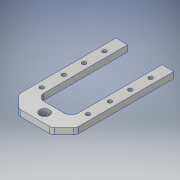
# Autodesk Inventor part: Part1_new1
Saved by Autodesk Inventor 2016 (Build 200138000, 138)
## iProperties
Created: 2017-01-04
Part Number: Part1_new1
Material: Aluminium 6061
Document SubType Name: Modeling
Designer: Marc
Density: 2.7 g/cm^3
Appearance: Aluminium - flach
Mass: 11.4747 g
Surface Area: 37.37 cm^2
Volume: 4.24988 cm^3
Author: Marc
Autodesk Inventor part; units mm, degrees
ref_plane "YZ Plane" through (0, 0, 0) normal (1, 0, 0) x (0, 1, 0)
ref_plane "XZ Plane" through (0, 0, 0) normal (0, 1, 0) x (-1, 0, 0)
ref_plane "XY Plane" through (0, 0, 0) normal (0, 0, 1) x (1, 0, 0)
sketch "Skizze2" plane through (0, 0, 0) normal (0, 0, 1) x (1, 0, 0)
  line L0 (-26.1954, 0) -> (26.1954, 0) projected
  line L1 (0, -30.2532) -> (0, 68.0422) projected
  line L2 (-18.5, 54) -> (-18.5, -6.7574)
  line L3 (-9.2574, -16) -> (9.2574, -16)
  line L4 (18.5, -6.7574) -> (18.5, 54)
  line L5 (18.5, 54) -> (11, 54)
  line L6 (11, 54) -> (11, 3)
  line L7 (-11, 3) -> (-11, 54)
  line L8 (-11, 54) -> (-18.5, 54)
  circle A0 centre (0, -10) radius 3.15
  circle A1 centre (-14.75, 43) radius 1.3
  circle A2 centre (-14.75, 30) radius 1.3
  circle A3 centre (-14.75, 17) radius 1.3
  circle A4 centre (-14.75, 3) radius 1.3
  circle A5 centre (14.75, 43) radius 1.3
  circle A6 centre (14.75, 30) radius 1.3
  circle A7 centre (14.75, 17) radius 1.3
  circle A8 centre (14.75, 3) radius 1.3
  line L9 (-17.6213, -8.8787) -> (-11.3787, -15.1213)
  line L10 (11.3787, -15.1213) -> (17.6213, -8.8787)
  arc A9 (-18.5, -6.7574) -> (-17.6213, -8.8787) centre (-15.5, -6.7574) ccw
  arc A10 (-11.3787, -15.1213) -> (-9.2574, -16) centre (-9.2574, -13) ccw
  arc A11 (9.2574, -16) -> (11.3787, -15.1213) centre (9.2574, -13) ccw
  line L11 (-11, 3) -> (-11, 0.2426)
  line L12 (11, 3) -> (11, 0.2426)
  line L13 (-6.7574, -4) -> (6.7574, -4)
  line L14 (-10.1213, -1.8787) -> (-8.8787, -3.1213)
  line L15 (8.8787, -3.1213) -> (10.1213, -1.8787)
  arc A12 (-11, 0.2426) -> (-10.1213, -1.8787) centre (-8, 0.2426) ccw
  arc A13 (-8.8787, -3.1213) -> (-6.7574, -4) centre (-6.7574, -1) ccw
  arc A14 (6.7574, -4) -> (8.8787, -3.1213) centre (6.7574, -1) ccw
  arc A15 (10.1213, -1.8787) -> (11, 0.2426) centre (8, 0.2426) ccw
  arc A16 (17.6213, -8.8787) -> (18.5, -6.7574) centre (15.5, -6.7574) ccw
  point P0 (0, 0)
  point P1 (-18.5, -16)
  point P2 (18.5, -16)
  point P3 (11, 0)
  point P4 (-11, 0)
  point P5 (-8, 0)
  point P6 (-11, 3)
  point P7 (8, 0)
  point P8 (11, 3)
  point P9 (-18.5, -8)
  point P10 (-10.5, -16)
  point P11 (10.5, -16)
  point P12 (18.5, -8)
  point P13 (-11, -4)
  point P14 (11, -4)
  point P15 (-11, -1)
  point P16 (-8, -4)
  point P17 (8, -4)
  point P18 (11, -1)
  dimension "d0" = 70
  dimension "d1" = 37
  dimension "d2" = 90
  dimension "d3" = 70
  dimension "d4" = 90
  dimension "d6" = 7.5
  dimension "d8" = 90
  dimension "d9" = 22
  dimension "d10" = 54
  dimension "d11" = 6.3
  dimension "d13" = 6
  dimension "d14" = 2.6
  dimension "d15" = 3.75
  dimension "d16" = 11
  dimension "d17" = 2.6
  dimension "d18" = 2.6
  dimension "d19" = 2.6
  dimension "d20" = 13
  dimension "d21" = 13
  dimension "d22" = 14
  dimension "d23" = 3.75
  dimension "d24" = 3.75
  dimension "d25" = 3.75
  dimension "d26" = 2.6
  dimension "d27" = 2.6
  dimension "d28" = 2.6
  dimension "d29" = 2.6
  dimension "d30" = 3.75
  dimension "d31" = 3
  dimension "d32" = 3
  dimension "d33" = 3
  dimension "d34" = 3
  dimension "d35" = 8
  dimension "d36" = 8
  dimension "d37" = 8
  dimension "d38" = 8
  dimension "d45" = 7
  dimension "d46" = 7
  dimension "d47" = 3
  dimension "d48" = 3
  dimension "d49" = 3
  dimension "d50" = 3
  dimension "d51" = 3
  dimension "d52" = 90
  dimension "d53" = 54
  dimension "d54" = 4
  dimension "d55" = 11
  dimension "d56" = 8
  dimension "d57" = 8
  dimension "d58" = 3
  constraints: 30 point on line, 28 end point, 17 centre point, 16 point on circle, 16 tangent, 6 equal radius, 5 perpendicular, 4 horizontal alignment, 3 vertical alignment, 1 horizontal, 1 parallel, 1 vertical, 1 other
  measures "d0" distance of L2.start point (-18.5, -16)
  measures "d1" distance of point (-18.5, -16) point (18.5, -16)
  measures "d2" angle of L3 L2
  measures "d3" distance of point (18.5, -16) L4.end
  measures "d4" angle of L4 L3
  measures "d6" distance of L4.end L5.end
  measures "d8" angle of L6 L5
  measures "d9" distance of point (11, 0) point (-11, 0)
  measures "d10" distance of point (-11, 0) L7.end
  measures "d11" diameter of A0
  measures "d13" distance from line of L3 A0.centre
  measures "d14" diameter of A1
  measures "d15" distance from line of L7 A1.centre
  measures "d16" distance from line of L8 A1.centre
  measures "d17" diameter of A2
  measures "d18" diameter of A3
  measures "d19" diameter of A4
  measures "d20" distance of A1.centre A2.centre
  measures "d21" distance of A3.centre A2.centre
  measures "d22" distance of A4.centre A3.centre
  measures "d23" distance from line of L7 A2.centre
  measures "d24" distance from line of L7 A3.centre
  measures "d25" distance from line of L7 A4.centre
  measures "d26" diameter of A5
  measures "d27" diameter of A6
  measures "d28" diameter of A7
  measures "d29" diameter of A8
  measures "d30" distance from line of L4 A5.centre
  measures "d31" distance of point (-8, 0) point (-11, 0)
  measures "d32" distance of point (-11, 3) point (-11, 0)
  measures "d33" distance of point (8, 0) point (11, 0)
  measures "d34" distance of point (11, 3) point (11, 0)
  measures "d35" distance of point (-18.5, -8) point (-18.5, -16)
  measures "d36" distance of point (-10.5, -16) point (-18.5, -16)
  measures "d37" distance of point (10.5, -16) point (18.5, -16)
  measures "d38" distance of point (18.5, -8) point (18.5, -16)
  measures "d45" distance of L7.start point (-11, -4)
  measures "d46" distance of L6.end point (11, -4)
  measures "d47" distance of point (-11, -1) point (-11, -4)
  measures "d48" distance of point (-8, -4) point (-11, -4)
  measures "d49" distance of point (8, -4) point (11, -4)
  measures "d50" distance of point (11, -1) point (11, -4)
  measures "d51" radius of A12
  measures "d52" angle of L0 L7
  measures "d53" distance between parallel lines of L0 L5
  measures "d54" distance between parallel lines of L13 L0
  measures "d55" distance between parallel lines of L11 L1
  measures "d56" distance from line of point (8, 0) L1
  measures "d57" distance from line of point (-8, 0) L1
  measures "d58" radius of A16
extrude "Extrusion1" add sketch "Skizze2" along normal blind 4 contours L2 L8 L7 L11 A12 L0 | L0 A12 L14 A13 L13 L1 A0 L3 A10 L9 A9 L2 | A15 L12 L6 L5 L4 L0 | L0 L4 A16 L10 A11 L3 L1 A0 L13 A14 L15 A15
equation "\"d3\" = d0"
equation "\"d14\" = d29"
equation "\"d17\" = d28"
equation "\"d18\" = d28"
equation "\"d19\" = d29"
equation "\"d23\" = d24"
equation "\"d24\" = d25"
equation "\"d25\" = d15"
equation "\"d26\" = d29"
equation "\"d27\" = d28"
equation "\"d28\" = d29"
equation "\"d30\" = d15"
equation "\"d32\" = d31"
equation "\"d33\" = d31"
equation "\"d34\" = d33"
equation "\"d36\" = d35"
equation "\"d37\" = d35"
equation "\"d38\" = d37"
equation "\"d46\" = d45"
equation "\"d48\" = d47"
equation "\"d49\" = d47"
equation "\"d50\" = d49"
